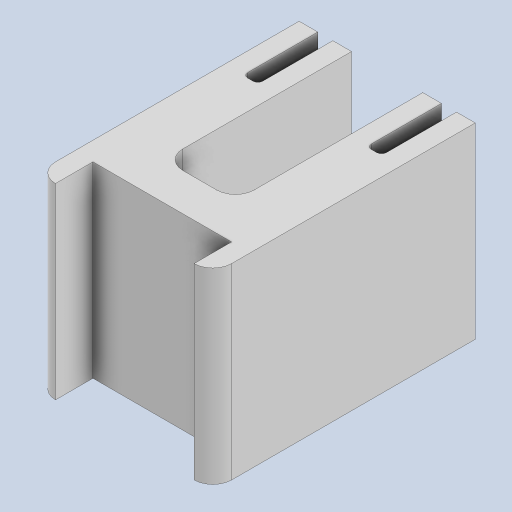
# Autodesk Inventor part: Sensore intermedio
Saved by Autodesk Inventor 2023.2 (Build 272271030, 271C)
## iProperties
Created: 2023-02-07
Part Number: Sensore intermedio
Material: Generico
Document SubType Name: Modeling
Designer: daler
Density: 1 g/cm^3
Appearance: Default
Author: daler
Autodesk Inventor part; units mm, degrees
ref_plane "YZ Plane" through (0, 0, 0) normal (1, 0, 0) x (0, 1, 0)
ref_plane "XZ Plane" through (0, 0, 0) normal (0, 1, 0) x (-1, 0, 0)
ref_plane "XY Plane" through (0, 0, 0) normal (0, 0, 1) x (1, 0, 0)
sketch "Schizzo1" plane through (0, 0, 0) normal (0, 0, 1) x (1, 0, 0)
  line L0 (-5.8, 10) -> (5.8, 10)
  line L1 (5.8, 10) -> (5.8, -10)
  line L2 (5.8, -10) -> (-5.8, -10)
  line L3 (-5.8, -10) -> (-5.8, 10)
  line L4 (-5.8, 10) -> (-7.4, 10)
  line L5 (-7.4, 10) -> (-7.4, -10)
  line L6 (-7.4, -10) -> (-5.8, -10)
  line L7 (-5.8, -10) -> (-5.8, 10)
  line L8 (0, 10) -> (0, -10) construction
  line L9 (-7.4, 10) -> (-9.4, 10)
  line L10 (-9.4, 10) -> (-9.4, -10)
  line L11 (-9.4, -10) -> (-7.4, -10)
  line L12 (-7.4, -10) -> (-7.4, 10)
  line L13 (-5.8, 0) -> (5.8, 0) construction
  line L14 (5.8, 10) -> (7.4, 10)
  line L15 (7.4, -10) -> (5.8, -10)
  line L16 (7.4, 10) -> (9.4, 10)
  line L17 (9.4, 10) -> (9.4, -10)
  line L18 (9.4, -10) -> (7.4, -10)
  line L19 (7.4, -10) -> (7.4, 10)
  line L20 (-3.8, -10) -> (-3.8, 10)
  line L21 (3.8, -10) -> (3.8, 10)
  point P0 (0, 0)
  point P1 (0, 0)
  point P2 (-5.8, -10)
  point P3 (-7.4, -10)
  point P4 (5.8, -10)
  point P5 (7.4, -10)
  point P6 (-5.8, -10)
  dimension "d1" = 20
  dimension "d2" = 1.6
  dimension "d3" = 2
  dimension "d6" = 2
  dimension "d7" = 2
  dimension "d20" = 7.6
  constraints: 44 end point, 6 parallel, 6 symmetric about line, 5 midpoint, 5 perpendicular, 4 point on line, 3 horizontal, 1 coincident
  measures "d1" distance of L0.end L1.end
  measures "d2" distance of L5.end L6.end
  measures "d3" distance of L4.end L9.end
  measures "d6" distance between parallel lines of L7 L20
  measures "d7" distance between parallel lines of L1 L21
  measures "d20" distance between parallel lines of L21 L20
extrude "Estrusione1" add sketch "Schizzo1" along normal blind 4
extrude "Estrusione2" add sketch "Schizzo1" against normal blind 20 contours L0 L20 L2 L3 | L5 L11 L10 L9 | L0 L1 L2 L21 | L16 L17 L18 L19
extrude "Estrusione3" add sketch "Schizzo1" against normal blind 12 contours L3 L6 L5 L4 | L14 L19 L15 L1
fillet "Raccordo1" radius 2 2 edges at (-3.8, 0, 0) (3.8, 0, 0)
sketch "Schizzo3" plane through (0, 0, 4) normal (0, 0, 1) x (1, 0, 0)
  line L0 (-9.4, 10) -> (-9.4, -10) projected
  line L1 (-9.4, -10) -> (9.4, -10) projected
  line L2 (-9.4, 10) -> (-7.4, 10)
  line L3 (-7.4, 10) -> (-7.4, -10)
  line L4 (-7.4, -10) -> (-9.4, -10)
  line L5 (-9.4, -10) -> (-9.4, 10)
  line L6 (9.4, 10) -> (7.4, 10)
  line L7 (7.4, 10) -> (7.4, -10)
  line L8 (7.4, -10) -> (9.4, -10)
  line L9 (9.4, -10) -> (9.4, 10)
  line L10 (9.4, -10) -> (9.4, 10) projected
  point P0 (0, 0)
  point P1 (9.4, 0)
  dimension "d16" = 2
  dimension "d17" = 2
  constraints: 16 end point, 4 parallel, 2 horizontal, 2 midpoint, 2 perpendicular, 2 point on line
  measures "d16" distance between parallel lines of L0 L3
  measures "d17" distance between parallel lines of L9 L7
extrude "Estrusione5" add sketch "Schizzo3" along normal blind 4
fillet "Raccordo3" radius 0.5 4 edges at (7.4, 0, -12) (5.8, 0, -12) (-7.4, 0, -12) (-5.8, 0, -12)
fillet "Raccordo4" radius 2 2 edges at (9.4, 0, 8) (-9.4, 0, 8)
